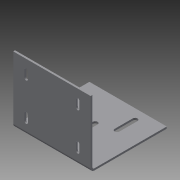
# Autodesk Inventor part: subframe
Saved by Autodesk Inventor 2014 SP2 (Build 180246200, 246)
## iProperties
Created: 2016-05-19
Part Number: subframe
Material: Generic
Document SubType Name: Sheet Metal
Designer: cruiser
Density: 1 g/cm^3
Sheet Metal Rule: Default_mm
Appearance: Default
Flat Pattern Width: 11.8828 cm
Flat Pattern Length: 6.6 cm
Flat Pattern Area: 78.4267 cm^2
Sheet Metal Width: 118.828 mm
Sheet Metal Length: 66.000 mm
Sheet Metal Area: 7842.670 mm^2
Author: cruiser
Autodesk Inventor part; units mm, degrees
ref_plane "YZ Plane" through (0, 0, 0) normal (1, 0, 0) x (0, 1, 0)
ref_plane "XZ Plane" through (0, 0, 0) normal (0, 1, 0) x (-1, 0, 0)
ref_plane "XY Plane" through (0, 0, 0) normal (0, 0, 1) x (1, 0, 0)
sketch "Sketch1" plane through (0, 0, 0) normal (0, 1, 0) x (-1, 0, 0)
  line L0 (33, -27.5) -> (-33, -27.5)
  line L1 (-33, -27.5) -> (-33, 27.5)
  line L2 (-33, 27.5) -> (33, 27.5)
  line L3 (33, 27.5) -> (33, -27.5)
  line L4 (33, -27.5) -> (-33, 27.5) construction
  line L5 (-33, -27.5) -> (33, 27.5) construction
  point P0 (0, 0)
  dimension "d0" = 66
  dimension "d1" = 55
  measures "d0" distance of L1.end L2.end
  measures "d1" distance of L0.end L1.end
extrude "Plate1" add sketch "Sketch1" along normal blind 1.5875
sketch "Sketch3" plane through (0, 1.5875, 0) normal (0, 1, 0) x (1, 0, 0)
  line L0 (0, 0) -> (-33, 0)
  line L1 (-33, 0) -> (-33, 27.5)
  line L2 (-33, 27.5) -> (0, 27.5)
  line L3 (0, 27.5) -> (0, 0)
  circle A0 centre (-22, 16) radius 1.5
  circle A1 centre (-22, -16) radius 1.5
  circle A2 centre (22, 16) radius 1.5
  circle A3 centre (22, -16) radius 1.5
  line L4 (-22, 13) -> (-22, 19) construction
  line L5 (-20.5, 13) -> (-20.5, 19)
  line L6 (-23.5, 19) -> (-23.5, 13)
  arc A4 (-23.5, 13) -> (-20.5, 13) centre (-22, 13) ccw
  arc A5 (-20.5, 19) -> (-23.5, 19) centre (-22, 19) ccw
  line L7 (20.5, 13) -> (20.5, 19)
  line L8 (23.5, 19) -> (23.5, 13)
  arc A6 (20.5, 13) -> (23.5, 13) centre (22, 13) ccw
  arc A7 (23.5, 19) -> (20.5, 19) centre (22, 19) ccw
  line L9 (-20.5, -13) -> (-20.5, -19)
  line L10 (-23.5, -19) -> (-23.5, -13)
  arc A8 (-20.5, -13) -> (-23.5, -13) centre (-22, -13) ccw
  arc A9 (-23.5, -19) -> (-20.5, -19) centre (-22, -19) ccw
  arc A10 (20.5, -19) -> (23.5, -19) centre (22, -19) ccw
  line L11 (23.5, -19) -> (23.5, -13)
  line L12 (20.5, -13) -> (20.5, -19)
  arc A11 (23.5, -13) -> (20.5, -13) centre (22, -13) ccw
  dimension "d22" = 3
  dimension "d23" = 32
  dimension "d24" = 22
  dimension "d48" = 3
  dimension "d49" = 3
  constraints: 28 end point, 21 symmetric about line, 16 point on circle, 12 centre point, 4 parallel, 4 tangent, 1 horizontal, 1 midpoint, 1 perpendicular, 9 other
  measures "d22" diameter of A0
  measures "d23" diameter of A0.centre L0
  measures "d24" distance from line of L3 A0.centre
  measures "d48" distance of A0.centre L4.end
  measures "d49" diameter of A5
extrude "Cut1" cut sketch "Sketch3" against normal blind 1.5875 contours A0 | L5 A4 L6 A0 | A0 L6 A5 L5 | A1 | L9 A9 L10 A1 | A1 L10 A8 L9 | A2 | L8 A6 L7 A2 | A2 L7 A7 L8 | A3 | L11 A10 L12 A3 | A3 L12 A11 L11
sketch "Sketch2" plane through (-33, 1.5875, -27.5) normal (0, 0, -1) x (-1, 0, 0)
  line L0 (-66, 0) -> (0, 0)
  line L1 (0, 0) -> (0, 63.4125)
  line L2 (0, 63.4125) -> (-66, 63.4125)
  line L3 (-66, 63.4125) -> (-66, 0)
  constraints: 6 end point, 1 horizontal, 1 perpendicular, 1 vertical
edge flange "Flange1" height 65 angle 90 thickness 1.5875 bend radius 1.5875 thickness toward (0, 0, -1) relief straight relief width 1.5875 relief depth 0.7937 edges at (0, 1.5875, -27.5) wall of the first edge with corners at (33, 1.5875, -27.5) (-33, 1.5875, -27.5) (-33, 65, -27.5) (33, 65, -27.5)
bend "Bend1"
corner "Corner1"
sketch "Sketch4" plane through (33, 65, -29.0875) normal (0, 0, -1) x (-1, 0, 0)
  line L0 (0, -61.825) -> (66, -61.825) projected
  line L1 (66, 0) -> (66, -61.825) projected
  line L2 (0, 0) -> (66, 0) projected
  line L3 (33, -34) -> (33, -28) construction
  line L4 (35, -34) -> (35, -28)
  line L5 (31, -28) -> (31, -34)
  arc A0 (31, -34) -> (35, -34) centre (33, -34) ccw
  arc A1 (35, -28) -> (31, -28) centre (33, -28) ccw
  line L6 (33, -61.825) -> (33, 0)
  line L7 (47.5, -24) -> (47.5, -8.5) construction
  line L8 (49.5, -24) -> (49.5, -8.5)
  line L9 (45.5, -8.5) -> (45.5, -24)
  arc A2 (45.5, -24) -> (49.5, -24) centre (47.5, -24) ccw
  arc A3 (49.5, -8.5) -> (45.5, -8.5) centre (47.5, -8.5) ccw
  line L10 (18.5, -24) -> (18.5, -8.5) construction
  line L11 (16.5, -24) -> (16.5, -8.5)
  line L12 (20.5, -8.5) -> (20.5, -24)
  arc A4 (16.5, -24) -> (20.5, -24) centre (18.5, -24) ccw
  arc A5 (20.5, -8.5) -> (16.5, -8.5) centre (18.5, -8.5) ccw
  line L13 (66, -65) -> (0, -65) projected
  point P0 (33, -65)
  point P1 (33, -31)
  point P2 (47.5, -16.25)
  point P3 (18.5, -16.25)
  dimension "d25" = 3
  dimension "d26" = 4
  dimension "d29" = 4
  dimension "d30" = 15.5
  dimension "d31" = 14.5
  dimension "d46" = 48.75
  dimension "d47" = 34
  constraints: 26 end point, 12 point on circle, 8 tangent, 7 symmetric about line, 6 centre point, 4 midpoint, 4 parallel, 1 point on line, 2 other
  measures "d25" distance of point (33, -31) L3.end
  measures "d26" diameter of A1
  measures "d29" diameter of A3
  measures "d30" distance of L7.start L7.end
  measures "d31" distance from line of L6 point (47.5, -16.25)
  measures "d46" distance from line of point (47.5, -16.25) L13
  measures "d47" distance from line of L13 point (33, -31)
extrude "Cut2" cut sketch "Sketch4" against normal blind 1.5875 contours L6 A1 L4 A0 | A0 L5 A1 L6 | L11 A5 L12 A4
equation "\"d0\" = subframe_x"
equation "\"d1\" = subframe_y"
equation "\"d22\" = m3_diameter"
equation "\"d23\" = 0.4 * frame_y"
equation "\"d24\" = 0.333333 * subframe_x"
equation "\"d49\" = m3_diameter"
equation "\"d20\" = Thickness"
equation "\"d26\" = m4_diameter"
equation "\"d29\" = m4_diameter"
equation "\"d33\" = Thickness"
equation "\"Thickness\" = sm_thickness"
equation "\"d3\" = BendReliefWidth"
equation "\"d4\" = BendReliefDepth"
equation "\"d5\" = MinimumRemnant"
equation "\"d6\" = BendRadius"
equation "\"d7\" = galvo_frame_z"
equation "\"d9\" = BendRadius"
equation "\"d11\" = CornerReliefSize"
equation "\"d12\" = GapSize"
equation "\"d13\" = JacobiRadiusSize"
equation "\"BendRadius\" = Thickness"
equation "\"BendReliefWidth\" = Thickness"
equation "\"BendReliefDepth\" = 0.5 * Thickness"
equation "\"CornerReliefSize\" = 4 * Thickness"
equation "\"MinimumRemnant\" = 2 * Thickness"
equation "\"TransitionRadius\" = BendRadius"
equation "\"JacobiRadiusSize\" = BendRadius"
equation "\"GapSize\" = Thickness"
equation "\"sm_thickness\" = 1.5875"
equation "\"very_thick_acrylic\" = 9.45"
equation "\"thick_acrylic\" = 5.88"
equation "\"thin_acrylic\" = 3.15"
equation "\"clear_acrylic\" = 3.15"
equation "\"wood_thickness\" = 6.72"
equation "\"m3_diameter\" = 3"
equation "\"m3_head\" = 6"
equation "\"m4_diameter\" = 4"
equation "\"m5_diameter\" = 5"
equation "\"m5_head\" = 10.3"
equation "\"brass_insert_drill\" = 4"
equation "\"m5_brass_insert_drill\" = 6.7"
equation "\"m3_press_nut_drill\" = 4.5"
equation "\"m5_press_nut_drill\" = 6.5"
equation "\"laser_body_diameter\" = 12"
equation "\"carrier_y\" = 251"
equation "\"carrier_z\" = 12"
equation "\"visor_x\" = 253.925"
equation "\"visor_y\" = 108.65"
equation "\"window_z\" = 332.225"
equation "\"window_y\" = 88.65"
equation "\"window_overlap\" = 48"
equation "\"acrylic_into_frame\" = 5"
equation "\"door_x\" = 251"
equation "\"door_z\" = 332.225"
equation "\"door_overlap\" = 48"
equation "\"reservoir_x\" = 201"
equation "\"reservoir_y\" = 201"
equation "\"linear_bearing_spacing\" = 271"
equation "\"tray_border\" = 25"
equation "\"tray_x\" = 251"
equation "\"tray_y\" = 251"
equation "\"bed_z\" = 25"
equation "\"crane_z2\" = 12"
equation "\"switch_spacing\" = 19"
equation "\"frame_top_z\" = 385"
equation "\"frame_bottom_z\" = 275"
equation "\"frame_total_z\" = 661.5875"
equation "\"frame_face_y\" = 45"
equation "\"frame_border\" = 48.0375"
equation "\"frame_foot_z\" = 12"
equation "\"frame_screw_from_center\" = 25"
equation "\"laser_y_offset\" = 19.4"
equation "\"laser_diameter\" = 12"
equation "\"laser_z_offset\" = 55"
equation "\"laser_y\" = 15"
equation "\"laser_z\" = 75"
equation "\"laser_gap\" = 1"
equation "\"subframe_x\" = 66"
equation "\"subframe_y\" = 55"
equation "\"galvo_frame_x\" = 66"
equation "\"galvo_frame_z\" = 65"
equation "\"galvo_frame_y_offset\" = 27.5"
equation "\"drawer_x\" = 257.3"
equation "\"drawer_y\" = 85.2375"
equation "\"drawer_z\" = 278.175"
equation "\"drawer_support_from_top\" = 48"
equation "\"drawer_screw_z\" = 145"
equation "\"drawer_screw_from_center\" = 55"
equation "\"nema17_x\" = 43"
equation "\"d2\" = BendRadius"
equation "\"d44\" = galvo_frame_x"
equation "\"al_thickness\" = 1.5875"
equation "\"rivet_diameter\" = 3.3"
equation "\"bend_factor\" = 2.26205"
equation "\"sm_bend\" = 3.591"
equation "\"al_bend\" = 3.591"
equation "\"frame_x\" = 353.375"
equation "\"carrier_z2\" = 25"
equation "\"carrier_y2\" = 76.825"
equation "\"frame_y\" = 80"
body "Solid1"
